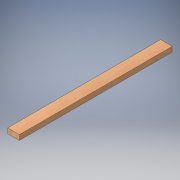
# Autodesk Inventor part: Lumbwer 2x4x50_75
Saved by Autodesk Inventor 2016 (Build 200138000, 138)
## iProperties
Created: 2015-05-31
Part Number: Lumbwer 2x4x50_75
Material: Wood (Birch)
Document SubType Name: Modeling
Designer: steele
Density: 0.55 g/cm^3
Appearance: Birch - Natural Polished
Author: steele
Autodesk Inventor part; units mm, degrees
ref_plane "YZ Plane" through (0, 0, 0) normal (1, 0, 0) x (0, 1, 0)
ref_plane "XZ Plane" through (0, 0, 0) normal (0, 1, 0) x (-1, 0, 0)
ref_plane "XY Plane" through (0, 0, 0) normal (0, 0, 1) x (1, 0, 0)
sketch "Sketch1" plane through (0, 0, 0) normal (0, 0, 1) x (1, 0, 0)
  line L0 (-44.45, -19.05) -> (44.45, -19.05)
  line L1 (44.45, -19.05) -> (44.45, 19.05)
  line L2 (44.45, 19.05) -> (-44.45, 19.05)
  line L3 (-44.45, 19.05) -> (-44.45, -19.05)
  line L4 (-44.45, -19.05) -> (44.45, 19.05) construction
  line L5 (44.45, -19.05) -> (-44.45, 19.05) construction
  point P0 (0, 0)
  dimension "d0" = 88.9
  dimension "d1" = 38.1
  constraints: 12 end point, 2 midpoint, 2 parallel, 1 horizontal, 1 perpendicular
  measures "d0" distance of L1.end L2.end
  measures "d1" distance of L0.end L1.end
extrude "Extrusion1" add sketch "Sketch1" along normal blind 1162.05
body "Solid1"
